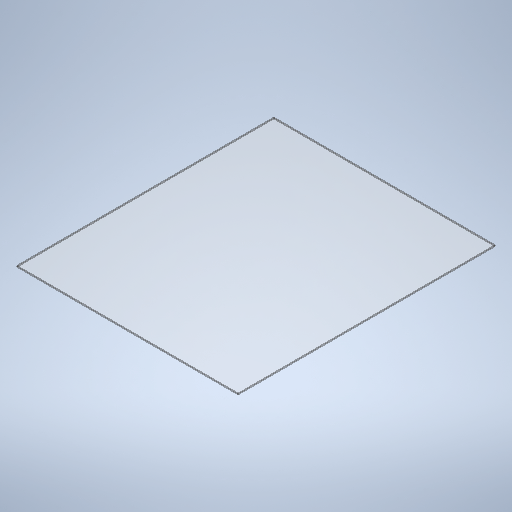
# Autodesk Inventor part: RT_FRM_V5_MC_01_DynamicsLeft
Saved by Autodesk Inventor 2025.3 (Build 293356000, 356)
## iProperties
Created: 2026-07-28
Part Number: RT_FRM_V5_MC_01_DynamicsLeft
Material: Polycarbonate, Clear
Document SubType Name: Modeling
Designer: louis
Density: 1.2 g/cm^3
Appearance: Polycarbonate - Clear
Author: louis
Autodesk Inventor part; units mm, degrees
ref_plane "YZ Plane" through (0, 0, 0) normal (1, 0, 0) x (0, 1, 0)
ref_plane "XZ Plane" through (0, 0, 0) normal (0, 1, 0) x (-1, 0, 0)
ref_plane "XY Plane" through (0, 0, 0) normal (0, 0, 1) x (1, 0, 0)
sketch "Sketch1" plane through (0, 0, 0) normal (0, 0, 1) x (1, 0, 0)
  line L0 (-310, -360) -> (310, -360)
  line L1 (310, -360) -> (310, 360)
  line L2 (310, 360) -> (-310, 360)
  line L3 (-310, 360) -> (-310, -360)
  line L4 (-310, -360) -> (310, 360) construction
  line L5 (310, -360) -> (-310, 360) construction
  point P0 (0, 0)
  dimension "d0" = 620
  dimension "d1" = 720
  constraints: 12 end point, 2 midpoint, 2 parallel, 1 horizontal, 1 perpendicular
  measures "d0" distance of L2.end L1.end
  measures "d1" distance of L1.end L0.end
extrude "Extrusion1" add sketch "Sketch1" against normal blind 3
body "Solid1"
